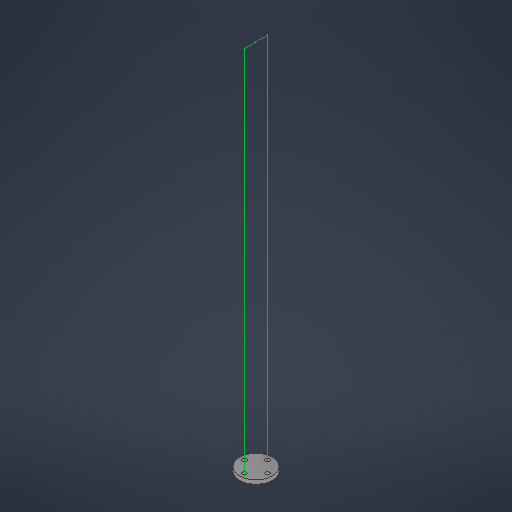
# Autodesk Inventor part: vakkarima
Saved by Autodesk Inventor 2026.1 (Build 301233020, 233B)
## iProperties
Created: 2025-10-06
Part Number: vakkarima
Material: Steel, Alloy
Document SubType Name: Modeling
Designer: Agi
Density: 7.73 g/cm^3
Appearance: Semi-Polished
Author: Agi
Autodesk Inventor part; units mm, degrees
ref_plane "YZ Plane" through (0, 0, 0) normal (1, 0, 0) x (0, 1, 0)
ref_plane "XZ Plane" through (0, 0, 0) normal (0, 1, 0) x (-1, 0, 0)
ref_plane "XY Plane" through (0, 0, 0) normal (0, 0, 1) x (1, 0, 0)
sketch "Sketch1" plane through (0, 0, 0) normal (1, 0, 0) x (0, 1, 0)
  line L0 (0, 0) -> (21, 0)
  line L1 (0, 0) -> (0, 39)
  line L2 (0, 39) -> (2, 39)
  line L3 (2, 39) -> (2, 70)
  line L4 (2, 70) -> (18, 70)
  line L5 (18, 70) -> (18, 0)
  dimension "d0" = 78
  dimension "d2" = 18
  dimension "d3" = 140
  dimension "d6" = 2
  constraints: 12 end point, 2 perpendicular, 1 horizontal, 1 point on line, 1 vertical
  measures "d0" diameter of L1.end L0
  measures "d2" horizontal distance of L4.end L1.end
  measures "d3" diameter of L4 L0
  measures "d6" distance between parallel lines of L1 L3
revolve "Revolution1" add sketch "Sketch1" angle 360 about axis through (0, 0, 0) along (0, 1, 0)
sketch "Sketch2" plane through (0, 18, 0) normal (0, 1, 0) x (1, 0, 0)
  point P0 (0, 0)
  point P1 (-50, 0)
  point P2 (0, 50)
  point P3 (50, 0)
  point P4 (0, -50)
hole "Hole1" at (-50, 18, 0) at (0, 18, -50) at (50, 18, 0) at (0, 18, 50) direction (0, -1, 0) diameter 18 end through all
fillet "Fillet1" radius 2 1 edges at (0, 2, -39)
body "Solid1"
